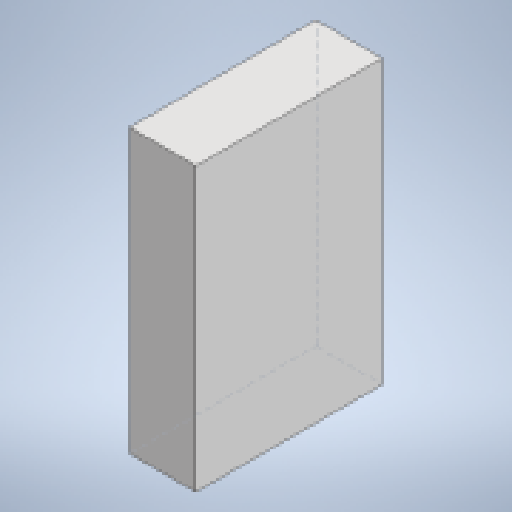
# Autodesk Inventor part: raspi
Saved by Autodesk Inventor 2023 (Build 270158000, 158)
## iProperties
Created: 2022-10-03
Part Number: raspi
Material: Polypropylene
Document SubType Name: Modeling
Designer: carso
Mass: 85.5848 g
Surface Area: 151.6 cm^2
Volume: 95.2 cm^3
Density: 0.899 g/cm^3
Appearance: Smooth - Ash
Author: carso
Autodesk Inventor part; units mm, degrees
ref_plane "YZ Plane" through (0, 0, 0) normal (1, 0, 0) x (0, 1, 0)
ref_plane "XZ Plane" through (0, 0, 0) normal (0, 1, 0) x (-1, 0, 0)
ref_plane "XY Plane" through (0, 0, 0) normal (0, 0, 1) x (1, 0, 0)
sketch "Sketch1" plane through (0, 0, 0) normal (1, 0, 0) x (0, 1, 0)
  line L0 (0, 0) -> (85, 0)
  line L1 (85, 0) -> (85, -56)
  line L2 (85, -56) -> (0, -56)
  line L3 (0, -56) -> (0, 0)
  dimension "d0" = 85
  dimension "d1" = 56
  constraints: 8 end point, 2 parallel, 1 horizontal, 1 perpendicular
  measures "d0" distance of L1.end L2.end
  measures "d1" distance of L0.end L1.end
extrude "Extrusion1" add sketch "Sketch1" along normal blind 20
sketch "Sketch2" plane through (0, 0, 0) normal (-1, 0, 0) x (0, 0, 1)
  line L0 (-3, 82) -> (-53, 82)
  line L1 (-53, 82) -> (-53, 3)
  line L2 (-53, 3) -> (-3, 3)
  line L3 (-3, 3) -> (-3, 82)
  line L4 (0, 0) -> (-56, 0) projected
  line L5 (0, 85) -> (0, 0) projected
  line L6 (-56, 85) -> (0, 85) projected
  line L7 (-56, 0) -> (-56, 85) projected
  line L8 (-53, 61) -> (-3, 61)
  dimension "d4" = 3
  dimension "d5" = 3
  dimension "d6" = 3
  dimension "d7" = 3
  dimension "d36" = 58
  constraints: 10 end point, 2 parallel, 2 perpendicular, 2 point on line, 1 horizontal
  measures "d4" distance between parallel lines of L4 L2
  measures "d5" distance between parallel lines of L5 L3
  measures "d6" distance between parallel lines of L6 L0
  measures "d7" distance between parallel lines of L7 L1
  measures "d36" distance between parallel lines of L2 L8
hole "Hole1" at (0, 3, -53) direction (1, 0, 0) diameter 2.7 depth 20
hole "Hole2" at (0, 3, -3) direction (1, 0, 0) diameter 2.7 depth 20
hole "Hole3" at (0, 82, -3) direction (1, 0, 0) diameter 2.7 depth 20
hole "Hole4" at (0, 82, -53) direction (1, 0, 0) diameter 2.7 depth 20
hole "Hole5" at (0, 61, -53) direction (1, 0, 0) diameter 2.7 depth 20
hole "Hole6" at (0, 61, -3) direction (1, 0, 0) diameter 2.7 depth 20
body "Solid1"
